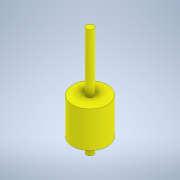
# Autodesk Inventor part: 1_Asse_cuscinetti
Saved by Autodesk Inventor 2020.2 (Build 242310000, 310)
## iProperties
Created: 2019-10-11
Part Number: 1_Asse_cuscinetti
Material: Asse pendolo
Document SubType Name: Modeling
Designer: socci
Density: 5.988 g/cm^3
Appearance: Giallo
Mass: 128.983 g
Surface Area: 52.0405 cm^2
Volume: 21.5403 cm^3
Author: socci
Autodesk Inventor part; units mm, degrees
ref_plane "YZ Plane" through (0, 0, 0) normal (1, 0, 0) x (0, 1, 0)
ref_plane "XZ Plane" through (0, 0, 0) normal (0, 1, 0) x (-1, 0, 0)
ref_plane "XY Plane" through (0, 0, 0) normal (0, 0, 1) x (1, 0, 0)
sketch "Schizzo1" plane through (0, 0, 0) normal (0, 1, 0) x (-1, 0, 0)
  circle A0 centre (0, 0) radius 14.5
  dimension "d0" = 29
  constraints: 1 centre point, 1 coincident
  measures "d0" diameter of A0
extrude "Estrusione1" add sketch "Schizzo1" along normal blind 30
sketch "Schizzo2" plane through (0, 0, 0) normal (0, -1, 0) x (1, 0, 0)
  circle A0 centre (0, 0) radius 3
  dimension "d3" = 6
  constraints: 1 centre point, 1 coincident
  measures "d3" diameter of A0
extrude "Estrusione2" add sketch "Schizzo2" along normal blind 12 and the other way blind 79
